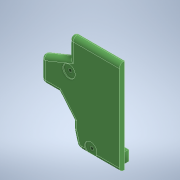
# Autodesk Inventor part: Top
Saved by Autodesk Inventor 2022 (Build 260153000, 153)
## iProperties
Created: 2023-08-27
Part Number: Top
Material: Типовые
Document SubType Name: Modeling
Designer: user
Density: 1 g/cm^3
Appearance: По умолчанию
Author: user
## iProperties of the stored document Top_3DПЕЧАТЬ.ipt
Created: 2023-08-30
Part Number: Top_3DПЕЧАТЬ
Material: Типовые
Document SubType Name: Modeling
Designer: user
Density: 1 g/cm^3
Appearance: По умолчанию
Author: user
Autodesk Inventor part; units mm, degrees
ref_plane "YZ Plane" through (0, 0, 0) normal (1, 0, 0) x (0, 1, 0)
ref_plane "XZ Plane" through (0, 0, 0) normal (0, 1, 0) x (-1, 0, 0)
ref_plane "XY Plane" through (0, 0, 0) normal (0, 0, 1) x (1, 0, 0)
sketch "Эскиз1" plane through (0, 0, 0) normal (0, 0, 1) x (1, 0, 0)
  line L0 (-41.7, -37.7) -> (-41.7, -22.5)
  line L1 (-41.7, -22.5) -> (-37.5, -22.5)
  line L2 (-37.5, -22.5) -> (-37.5, -24.2)
  line L3 (-37.5, -24.2) -> (-27.2, -24.2)
  line L4 (-27.2, -24.2) -> (-27.2, -22.5)
  line L5 (-27.2, -22.5) -> (-25, -22.5)
  line L6 (-25, -22.5) -> (-25, -24.2)
  line L7 (-25, -24.2) -> (-22.5, -24.2)
  line L8 (-22.5, -24.2) -> (-22.5, -61.2)
  line L9 (-22.5, -61.2) -> (-25, -61.2)
  line L10 (-25, -61.2) -> (-25, -62.9)
  line L11 (-25, -62.9) -> (-40, -62.9)
  line L12 (-40, -62.9) -> (-40, -55.0851)
  line L13 (-44.2, -20) -> (-20, -20)
  line L14 (-20, -20) -> (-20, -65.4)
  line L15 (-60, -70) -> (-20, -70)
  line L16 (-20, -65.4) -> (-42.5, -65.4)
  line L17 (-41.7, -37.7) -> (-55.2, -37.7)
  line L18 (-44.2, -20) -> (-44.2, -29.7)
  line L19 (-55.2, -37.7) -> (-55.2, -44.1)
  line L20 (-44.2, -29.7) -> (-57.7, -35.2)
  line L21 (-57.7, -35.2) -> (-57.7, -46.6)
  line L22 (-60, -20) -> (-60, -70)
  line L23 (-42.5, -65.4) -> (-42.5, -54.6)
  line L24 (-55.2, -44.1) -> (-53.2, -44.1)
  line L25 (-53.2, -44.1) -> (-53.2, -46.6)
  line L26 (-53.2, -46.6) -> (-57.7, -46.6)
  line L27 (-49.2, -44.1) -> (-49.2, -46.6)
  line L28 (-49.2, -46.6) -> (-42.5, -54.6)
  line L29 (-49.2, -44.1) -> (-40, -55.0851)
  line L30 (-49.2, -44.1) -> (-46.2, -44.1)
  line L31 (-46.2, -44.1) -> (-46.2, -47.6821)
  line L32 (-25, -62.9) -> (-22.5, -65.4)
  line L33 (-30, -62.9) -> (-32.5, -65.4)
  line L34 (-46.2, -44.1) -> (-46.2, -37.7)
  line L35 (-20, -70) -> (-20, -20)
  line L36 (-20, -20) -> (-60, -20)
  line L37 (-53.2, -46.6) -> (-49.2, -46.6)
  line L38 (-53.2, -44.1) -> (-55.7, -46.6)
  line L39 (-49.2, -44.1) -> (-46.7, -49.5851)
  circle A0 centre (-54.1298, -30.506) radius 0.8
  circle A1 centre (-54.1298, -30.506) radius 3
  line L40 (-55.7762, -34.4162) -> (-56.908, -31.6379)
  line L41 (-50.2196, -32.1524) -> (-51.3515, -29.3742)
  circle A2 centre (-33.7426, -62.4) radius 0.8
  circle A3 centre (-33.7426, -62.4) radius 3
  line L42 (-29, -50.4) -> (-26, -50.4)
  line L43 (-26, -50.4) -> (-26, -60.4)
  line L44 (-26, -60.4) -> (-29, -60.4)
  line L45 (-29, -60.4) -> (-29, -50.4)
  circle A4 centre (-44.2, -35.2) radius 0.8
  circle A5 centre (-44.2, -35.2) radius 3
  line L46 (-40.5725, -65.4) -> (-42.5, -58.2063)
  point P0 (0, 0)
  point P1 (-44.2, -20)
  point P2 (-42.5417, -37.7)
  point P3 (-41.7, -36.8583)
  point P4 (-41.7, -33.5417)
  point P5 (-45.8583, -37.7)
  dimension "d0" = 16.7
  dimension "d1" = 4.2
  dimension "d2" = 2.2
  dimension "d3" = 1.7
  dimension "d4" = 40.4
  dimension "d5" = 1.7
  dimension "d6" = 2.5
  dimension "d7" = 15
  dimension "d8" = 2.5
  dimension "d9" = 2.5
  dimension "d10" = 2.5
  dimension "d11" = 15.2
  dimension "d12" = 2.5
  dimension "d14" = 2.5
  dimension "d15" = 2.5
  dimension "d16" = 8
  dimension "d17" = 2.5
  dimension "d18" = 6.4
  dimension "d19" = 2.5
  dimension "d20" = 2
  dimension "d21" = 4
  dimension "d22" = 2.5
  dimension "d23" = 3
  dimension "d24" = 5
  dimension "d25" = 2.5
  dimension "d26" = 8
  dimension "d27" = 2.5
  dimension "d28" = 2.5
  dimension "d29" = 2.5
  dimension "d30" = 20
  dimension "d31" = 20
  dimension "d32" = 50
  dimension "d33" = 40
  dimension "d44" = 37.7
  dimension "d55" = 1.6
  dimension "d57" = 6
  dimension "d58" = 6.5
  dimension "d60" = 1.6
  dimension "d61" = 6
  dimension "d66" = 6
  dimension "d67" = 9
  dimension "d68" = 5
  dimension "d69" = 15
  dimension "d77" = 1.6
  dimension "d78" = 6
  dimension "d80" = 15.2
  dimension "d81" = 24.2
  dimension "d83" = 15
  dimension "d84" = 1.2
  constraints: 94 end point, 17 point on line, 13 perpendicular, 7 horizontal, 6 centre point, 5 parallel, 5 tangent, 5 vertical, 3 coincident, 3 collinear, 2 point on circle
  measures "d0" distance between parallel lines of L0 L6
  measures "d1" distance between parallel lines of L2 L0
  measures "d2" distance between parallel lines of L4 L6
  measures "d3" distance between parallel lines of L7 L5
  measures "d4" distance between parallel lines of L11 L5
  measures "d5" distance between parallel lines of L11 L9
  measures "d6" distance between parallel lines of L8 L6
  measures "d7" distance between parallel lines of L10 L12
  measures "d8" distance between parallel lines of L5 L13
  measures "d9" distance between parallel lines of L14 L8
  measures "d10" distance between parallel lines of L16 L11
  measures "d11" distance between parallel lines of L1 L17
  measures "d12" distance between parallel lines of L18 L0
  measures "d14" distance between parallel lines of L21 L19
  measures "d15" distance from line of L17 L21.start
  measures "d16" distance from line of L17 L18.end
  measures "d17" distance between parallel lines of L12 L23
  measures "d18" distance from line of L24.start L17
  measures "d19" horizontal distance of L26.end L24.start
  measures "d20" distance of L24.start L24.end
  measures "d21" distance between parallel lines of L27 L25
  measures "d22" distance of L27.end L29.start
  measures "d23" distance of L29.start L31.start
  measures "d24" distance from line of L33.start L10
  measures "d25" horizontal distance of L33.start L33.end
  measures "d26" distance from line of L28.end L26
  measures "d27" distance from line of L10 L32.end
  measures "d28" distance from line of L25 L38.end
  measures "d29" distance from line of L39.end L27
  measures "d30" distance from line of point (0, 0) L36
  measures "d31" distance from line of point (0, 0) L35
  measures "d32" distance between parallel lines of L36 L15
  measures "d33" distance between parallel lines of L35 L22
  measures "d44" distance between parallel lines of L35 L21
  measures "d55" diameter of A0
  measures "d57" diameter of A1
  measures "d58" distance from line of L18.end L41
  measures "d60" diameter of A2
  measures "d61" diameter of A3
  measures "d66" distance between parallel lines of L14 L43
  measures "d67" distance between parallel lines of L35 L45
  measures "d68" distance between parallel lines of L44 L16
  measures "d69" distance between parallel lines of L16 L42
  measures "d77" diameter of A4
  measures "d78" diameter of A5
  measures "d80" distance from line of A4.centre L36
  measures "d81" distance from line of L35 A4.centre
  measures "d83" angle of L46 L23
  measures "d84" distance from line of L11.end L46
extrude "Выдавливание1" add sketch "Эскиз1" along normal blind 2.5 contours L17 A5 L0 | L0 A5 L1 L2 L3 L4 L5 L6 L7 L8 L9 L10 L11 A3 L12 L29 L31 L34 L17 | A5 L17 L0 | L0 A5 | A5 L17 | A5 L17 L19 L24 L38 L26 L21 L20 L18 L13 L14 L16 L32 L10 L9 L8 L7 L6 L5 L4 L3 L2 L1 L0 | L34 L30 L27 L37 L25 L24 L19 L17 | L31 L29 L30 | L39 L28 L27 | L29 L12 L11 A3 L16 L46 L23 L28 L39 | L25 L26 L38 | A3 L11 A2 | L11 A2 A3 | A3 L33 L16 | L11 L33 A3 | L33 L11 L32 L16 | L42 L43 L44 L45
extrude "Выдавливание3" add sketch "Эскиз1" against normal blind 7 contours L33 L11 L32 L16
chamfer "Фаска1" distance 2.5 angle 45 1 edges at (-27.5, -65.4, -7)
fillet "Сопряжение1" radius 2 12 edges at (-44.2, -24.85, 2.5) (-50.95, -32.45, 2.5) (-57.7, -40.9, 2.5) (-53.45, -46.6, 2.5) (-45.85, -50.6, 2.5) (-42.5, -56.4032, 2.5) (-30.2862, -65.4, 2.5) (-57.7, -46.6, 1.25) (-57.7, -35.2, 1.25) (-32.1, -20, 2.5) (-44.2, -20, 1.25) (-41.5362, -61.8032, 2.5)
extrude "Выдавливание4" cut sketch "Эскиз1" against normal blind 0.5 from surface at 2.5 contours A5 L17 L0 | L0 A5 | A5 L17 | A3 L11 A2 | L11 A2 A3 picked at (-44.1679, -37.1314)
extrude "Выдавливание5" cut sketch "Эскиз1" along normal blind 1.5 contours L42 L43 L44 L45
fillet "Сопряжение3" radius 1 4 edges at (-29, -55.4, 0) (-27.5, -50.4, 0) (-26, -55.4, 0) (-27.5, -60.4, 0)
fillet "Сопряжение4" radius 3 2 edges at (-40.5725, -65.4, 0.25) (-40.123, -64.8142, 1.9142)
